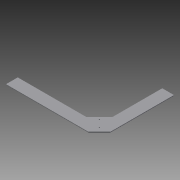
# Autodesk Inventor part: OptiTrack_Calibrator
Saved by Autodesk Inventor 2013 (Build 170138000, 138)
## iProperties
Created: 2015-03-28
Part Number: OptiTrack_Calibrator
Material: Generic
Document SubType Name: Modeling
Designer: Pat
Density: 1 g/cm^3
Author: Pat
Autodesk Inventor part; units mm, degrees
ref_plane "YZ Plane" through (0, 0, 0) normal (1, 0, 0) x (0, 1, 0)
ref_plane "XZ Plane" through (0, 0, 0) normal (0, 1, 0) x (-1, 0, 0)
ref_plane "XY Plane" through (0, 0, 0) normal (0, 0, 1) x (1, 0, 0)
sketch "Sketch1" plane through (0, 0, 0) normal (0, 1, 0) x (-1, 0, 0)
  line L0 (0, -232.2291) -> (0, -361.7009)
  line L1 (0, -361.7009) -> (63.5, -361.7009)
  line L2 (63.5, -361.7009) -> (63.5, -95.0009)
  line L3 (63.5, -95.0009) -> (135.342, -23.1589)
  line L4 (135.342, -23.1589) -> (503.642, -23.1589)
  line L5 (503.642, -23.1589) -> (503.642, 40.3411)
  line L6 (503.642, 40.3411) -> (59.142, 40.3411)
  line L7 (59.142, 40.3411) -> (0, -18.8009)
  line L8 (0, -18.8009) -> (0, -232.2291)
  line L9 (99.421, -59.0799) -> (29.571, 10.7701) construction
  circle A0 centre (86.8487, -46.5075) radius 2.54
  circle A1 centre (50.9276, -10.5865) radius 2.54
  point P0 (0, 0)
  dimension "d0" = 63.5
  dimension "d2" = 63.5
  dimension "d3" = 101.6
  dimension "d4" = 266.7
  dimension "d5" = 368.3
  dimension "d6" = 342.9
  dimension "d7" = 444.5
  dimension "d10" = 5.08
  dimension "d11" = 17.78
  dimension "d12" = 5.08
  dimension "d13" = 68.58
  constraints: 20 end point, 3 parallel, 3 perpendicular, 2 centre point, 2 midpoint, 2 point on line, 1 collinear, 1 vertical
  measures "d0" distance of L0.end L1.end
  measures "d2" distance of L4.end L5.end
  measures "d3" distance of L2.end L3.end
  measures "d4" distance of L1.end L2.end
  measures "d5" distance of L3.end L4.end
  measures "d6" distance of L7.end L0.end
  measures "d7" distance of L5.end L6.end
  measures "d10" diameter of A0
  measures "d11" distance from line of A0.centre L3
  measures "d12" diameter of A1
  measures "d13" distance from line of A1.centre L3
extrude "Extrusion1" add sketch "Sketch1" along normal blind 3.4925
body "Solid1"
